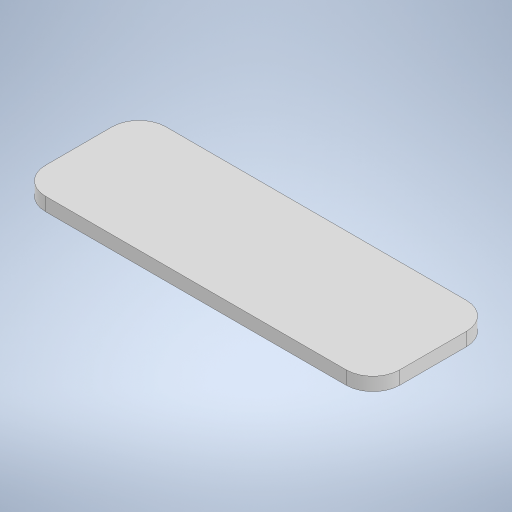
# Autodesk Inventor part: Pojemnik-Silnik
Saved by Autodesk Inventor 2023 (Build 270158000, 158)
## iProperties
Created: 2023-01-05
Part Number: Pojemnik-Silnik
Material: Ogólny
Document SubType Name: Modeling
Designer: User
Density: 1 g/cm^3
Appearance: Domyślna
Author: User
Autodesk Inventor part; units mm, degrees
ref_plane "YZ Plane" through (0, 0, 0) normal (1, 0, 0) x (0, 1, 0)
ref_plane "XZ Plane" through (0, 0, 0) normal (0, 1, 0) x (-1, 0, 0)
ref_plane "XY Plane" through (0, 0, 0) normal (0, 0, 1) x (1, 0, 0)
sketch "Szkic2" plane through (0, 0, 0) normal (0, 1, 0) x (-1, 0, 0)
  line L0 (6, 4.5) -> (-6, 4.5)
  line L1 (-6, 4.5) -> (-6, -4.5)
  line L2 (-6, -4.5) -> (6, -4.5)
  line L3 (6, -4.5) -> (6, 4.5)
  line L4 (9.7936, 0) -> (-12.3472, 0)
  line L5 (0, 10.0787) -> (0, -13.253)
  line L6 (6, 4.5) -> (11.25, 4.5)
  line L7 (13.25, 2.5) -> (13.25, -2.5)
  line L8 (11.25, -4.5) -> (6, -4.5)
  line L9 (6, -4.5) -> (6, 4.5)
  arc A0 (13.25, 2.5) -> (11.25, 4.5) centre (11.25, 2.5) ccw
  arc A1 (11.25, -4.5) -> (13.25, -2.5) centre (11.25, -2.5) ccw
  line L10 (-6, 4.5) -> (-11.25, 4.5)
  line L11 (-13.25, 2.5) -> (-13.25, -2.5)
  line L12 (-11.25, -4.5) -> (-6, -4.5)
  arc A2 (-11.25, 4.5) -> (-13.25, 2.5) centre (-11.25, 2.5) ccw
  arc A3 (-13.25, -2.5) -> (-11.25, -4.5) centre (-11.25, -2.5) ccw
  point P0 (0, 0)
  point P1 (13.25, 4.5)
  dimension "d7" = 12
  dimension "d8" = 9
  dimension "d9" = 4.5
  dimension "d10" = 6
  dimension "d11" = 7.25
  dimension "d12" = 2
  constraints: 26 end point, 8 point on circle, 7 symmetric about line, 4 centre point, 4 horizontal, 4 parallel, 4 tangent, 2 perpendicular, 2 point on line, 2 vertical, 1 equal radius, 2 other
  measures "d7" distance of L0.start L0.end
  measures "d8" distance of L2.end L0.start
  measures "d9" distance between parallel lines of L4 L0
  measures "d10" distance between parallel lines of L5 L3
  measures "d11" distance of L0.start point (13.25, 4.5)
  measures "d12" radius of A0
extrude "Wyciągnięcie proste2" add sketch "Szkic2" along normal blind 1
